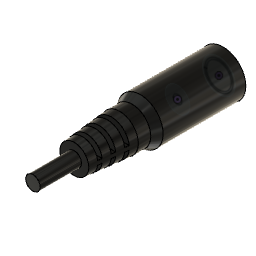
CircuitBox_cover_v10 (Autodesk Fusion 360 archive; units mm, degrees)
design "Power Plug"
Autodesk Fusion 360 part; units mm, degrees
sketch "Sketch1" plane through (0, 0, 0) normal (0, 1, 0) x (1, 0, 0)
  circle A0 centre (0, 0) radius 5.5
  dimension "d1" = 11
  constraint coincident A0.centre origin
  measures "d1" diameter of A0
ref_plane "WorkPlane1" through (0, 20, 0) normal (0, 1, 0) x (1, 0, 0)
sketch "Sketch2" plane through (0, 20, 0) normal (0, 1, 0) x (1, 0, 0)
  circle A0 centre (0, 0) radius 5.5
  dimension "d3" = 11
  constraint coincident A0.centre origin
  measures "d3" diameter of A0
ref_plane "WorkPlane2" through (0, -2, 0) normal (0, 1, 0) x (1, 0, 0)
sketch "Sketch3" plane through (0, -2, 0) normal (0, 1, 0) x (1, 0, 0)
  circle A0 centre (0, 0) radius 4.5
  dimension "d5" = 9
  constraint coincident A0.centre origin
  measures "d5" diameter of A0
ref_plane "WorkPlane3" through (0, -5, 0) normal (0, 1, 0) x (1, 0, 0)
sketch "Sketch4" plane through (0, -5, 0) normal (0, 1, 0) x (1, 0, 0)
  circle A0 centre (0, 0) radius 4.5
  dimension "d7" = 9
  constraint coincident A0.centre origin
  measures "d7" diameter of A0
ref_plane "WorkPlane4" through (0, -16, 0) normal (0, 1, 0) x (1, 0, 0)
sketch "Sketch5" plane through (0, -16, 0) normal (0, 1, 0) x (1, 0, 0)
  circle A0 centre (0, 0) radius 3.5
  dimension "d9" = 7
  constraint coincident A0.centre origin
  measures "d9" diameter of A0
loft "Loft1" add profiles "Sketch2", "Sketch1" section 1 section 2 makes body 1
loft "Loft2" add profiles "Sketch3" section 1 face at (-1.4907, 0, -0.2732) section 2 on bodies 1 bodies 1
loft "Loft3" add profiles "Sketch4" section 1 face at (0.9352, -2, -1.1727) section 2 on bodies 1 bodies 1
loft "Loft4" add profiles "Sketch5" section 1 face at (0.9352, -5, -1.1727) section 2 on bodies 1 bodies 1
sketch "Sketch6" plane through (0, 0, 0) normal (1, 0, 0) x (0, 1, 0)
  line L0 (-10.5, 5.5424) -> (-10.5, -7.5313)
  line L1 (-5, 0.5) -> (-16, 0.5)
  line L2 (-16, 0.5) -> (-16, -0.5)
  line L3 (-16, -0.5) -> (-5, -0.5)
  line L4 (-5, -0.5) -> (-5, 0.5)
  line L5 (-5, 0.5) -> (-16, -0.5) construction
  line L6 (-16, 0.5) -> (-5, -0.5) construction
  line L7 (-14, 5) -> (-13, 5)
  line L8 (-13, 5) -> (-13, -5)
  line L9 (-13, -5) -> (-14, -5)
  line L10 (-14, -5) -> (-14, 5)
  line L11 (-11, 5) -> (-10, 5)
  line L12 (-10, 5) -> (-10, -5)
  line L13 (-10, -5) -> (-11, -5)
  line L14 (-11, -5) -> (-11, 5)
  line L15 (-8, 5) -> (-7, 5)
  line L16 (-7, 5) -> (-7, -5)
  line L17 (-7, -5) -> (-8, -5)
  line L18 (-8, -5) -> (-8, 5)
  point P0 (-10.5, 0)
  point P1 (-10.5, 0)
  dimension "d10" = 11
  dimension "d11" = 1
  constraint horizontal L1
  constraint perpendicular L1 L2
  constraint parallel L1 L3
  constraint parallel L2 L4
  constraint coincident L5 P1
  constraint coincident L6 P1
  constraint coincident P0 P1
  constraint horizontal L7
  constraint vertical L8
  constraint horizontal L9
  constraint vertical L10
  constraint horizontal L11
  constraint vertical L12
  constraint horizontal L13
  constraint vertical L14
  constraint horizontal L15
  constraint vertical L16
  constraint horizontal L17
  constraint vertical L18
  measures "d10" distance of L2.end L3.end
  measures "d11" distance of L1.end L2.end
extrude "Extrude1" cut sketch "Sketch6" along normal blind 5 and the other way blind 5 contours L0 L1 L11 L12 | L0 L1 L11 L14 | L0 L3 L12 L13 | L0 L3 L13 L14 | L1 L15 L16 L18 | L1 L7 L8 L10 | L3 L8 L9 L10 | L3 L16 L17 L18 bodies 1
sketch "Sketch7" plane through (0, -16, 0) normal (0, -1, 0) x (1, 0, 0)
  circle A0 centre (0, 0) radius 3.5
  circle A1 centre (0, 0) radius 1.75
  dimension "d16" = 3.5
  constraint concentric A0 A1
  measures "d16" diameter of A1
extrude "Extrude2" add sketch "Sketch7" against normal blind 11 contours A1 bodies 1
sketch "Sketch8" plane through (0, 20, 0) normal (0, 1, 0) x (-1, 0, 0)
  circle A0 centre (0, 0) radius 5.5
  circle A1 centre (0, 0) radius 4
  dimension "d19" = 8
  constraint coincident A0.centre A1.centre
  measures "d19" diameter of A1
extrude "Extrude3" cut sketch "Sketch8" against normal blind 1 contours A1 bodies 1
sketch "Sketch9" plane through (0, 19, 0) normal (0, 1, 0) x (-1, 0, 0)
  circle A0 centre (0, 0) radius 4
  circle A1 centre (0, 0) radius 3
  circle A2 centre (0, 0) radius 3.4
  dimension "d22" = 6
  dimension "d23" = 6.8
  constraint coincident A0.centre A1.centre
  measures "d22" diameter of A1
  measures "d23" diameter of A2
extrude "Extrude4" cut sketch "Sketch9" against normal blind 10 bodies 1
sketch "Sketch10" plane through (0, 9, 0) normal (0, 1, 0) x (-1, 0, 0)
  circle A0 centre (0, 0) radius 3
  circle A1 centre (0, 0) radius 1
  dimension "d26" = 2
  constraint coincident A0.centre A1.centre
  measures "d26" diameter of A1
extrude "Extrude5" add sketch "Sketch10" along normal blind 9 contours A1 bodies 1
fillet "Fillet1" radius 0.8 1 edges at (0.9323, 18, -0.3616) on bodies 1
extrude "Extrude6" add sketch "Sketch7" along normal blind 10 contours A1 bodies 1
copy_body "Body->Comp1" bodies 1 removing the originals makes body 2 in component "Component"
sketch "Sketch11" plane through (0, 0, 0) normal (0, 0, 1) x (1, 0, 0)
  line L0 (10, 20) -> (43, 20)
  line L1 (43, 20) -> (43, -16)
  line L2 (43, -16) -> (10, -16)
  line L3 (10, -16) -> (10, 20)
  constraint horizontal L0
  constraint vertical L1
  constraint horizontal L2
  constraint vertical L3
component "Component" placed x (1, 0, 0) y (0, 1, 0) z (0, 0, 1) at (0, 0, 0)
